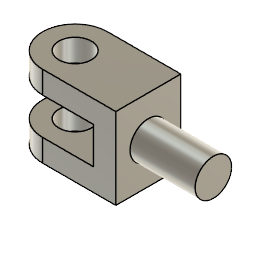
EDM EX 3.1 (Autodesk Fusion 360 design; units mm, degrees)
part number: 2025-10-06-08-14-35-849
Autodesk Fusion 360 part; units mm, degrees
note: some values were not read from the file. Set by a fixed rule: which sketch regions a step uses.
sketch "Sketch1" plane through (0, 0, 0) normal (0, 0, 1) x (1, 0, 0)
  circle A0 centre (0, 0) radius 8
  line L0 (0, 16) -> (36, 16)
  line L1 (36, 16) -> (36, -16)
  line L2 (36, -16) -> (0, -16)
  arc A1 (0, 16) -> (0, -16) centre (0, 0) ccw
  dimension "d1" = 16
  dimension "d2" = 32
  dimension "d3" = 36
  dimension "d4" = 32
  constraint coincident A0.centre A1.centre
  constraint horizontal L0
  constraint vertical L1
  constraint horizontal L2
  measures "d1" diameter of A0
  measures "d2" diameter of A1
  measures "d3" distance of L0.start L0.end
  measures "d4" distance of L0.start L2.end
extrude "Extrude1" add sketch "Sketch1" along normal blind 11
sketch "Sketch2" plane through (0, 0, 11) normal (0, 0, 1) x (-1, 0, 0)
  circle A0 centre (0, 0) radius 8
  line L0 (-36, -16) -> (0, -16)
  arc A1 (0, -16) -> (0, 16) centre (0, 0) ccw
  line L1 (0, 16) -> (-36, 16)
  line L2 (-36, 16) -> (-36, -16)
  line L3 (-36, -16) -> (-25, -16)
  line L4 (-25, -16) -> (-25, 16)
  line L5 (-25, 16) -> (-36, 16)
  line L6 (-36, 16) -> (-36, -16)
  dimension "d7" = 11
  dimension "d8" = 32
  constraint horizontal L3
  constraint vertical L4
  constraint horizontal L5
  constraint vertical L6
  constraint coincident L0.start L2.end
  measures "d7" distance of L0.start L3.end
  measures "d8" distance of L0.start L1.end
extrude "Extrude2" add sketch "Sketch2" along normal blind 18 contours L0 L1 L2 L3 L4 L5 L6
sketch "Sketch3" plane through (0, 0, 29) normal (0, 0, 1) x (-1, 0, 0)
  line L0 (-36, 16) -> (-36, -16)
  line L1 (-36, -16) -> (-25, -16)
  line L2 (-25, -16) -> (-25, 16)
  line L3 (-25, 16) -> (-36, 16)
  line L4 (-36, -16) -> (0, -16)
  line L5 (0, -16) -> (0, 16)
  line L6 (0, 16) -> (-36, 16)
  line L7 (-36, 16) -> (-36, -16)
  circle A0 centre (0, 0) radius 8
  circle A1 centre (0, 0) radius 16
  dimension "d11" = 36
  dimension "d12" = 32
  dimension "d13" = 16
  dimension "d14" = 32
  constraint horizontal L4
  constraint vertical L5
  constraint horizontal L6
  constraint vertical L7
  constraint coincident L0.end L1.start
  constraint coincident A0.centre A1.centre
  constraint concentric A0 A1
  measures "d11" distance of L0.end L4.end
  measures "d12" distance of L0.end L0.start
  measures "d13" diameter of A0
  measures "d14" diameter of A1
extrude "Extrude3" add sketch "Sketch3" along normal blind 11 contours L0 L1 L2 L3 L4 L6 L7 | L2 L4 L6 A1 | L5 A0 A1 | L5 A0 A1
sketch "Sketch4" plane through (36, 0, 0) normal (1, 0, 0) x (0, 1, 0)
  line L0 (-16, 0) -> (16, 0)
  line L1 (16, 0) -> (16, 40)
  line L2 (16, 40) -> (-16, 40)
  line L3 (-16, 40) -> (-16, 0)
  line L4 (16, 0) -> (16, 20)
  line L5 (16, 20) -> (0, 20)
  circle A0 centre (0, 20) radius 9
  dimension "d17" = 20
  dimension "d18" = 16
  dimension "d19" = 18
  constraint coincident L0.end L1.start
  constraint perpendicular L0 L4
  constraint perpendicular L4 L5
  constraint coincident L5.end A0.centre
  measures "d17" distance of L0.end L4.end
  measures "d18" distance of L4.end L5.end
  measures "d19" diameter of A0
extrude "Extrude4" add sketch "Sketch4" along normal blind 32 contours A0
